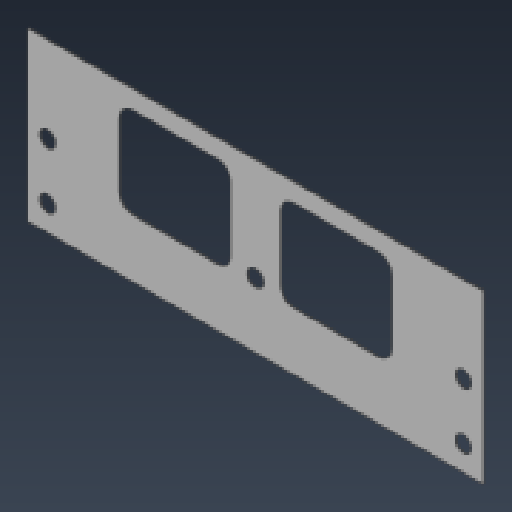
# Autodesk Inventor part: spring_steel_front
Saved by Autodesk Inventor 2023 (Build 270158000, 158)
## iProperties
Created: 2026-01-11
Part Number: spring_steel_front
Material: Steel
Document SubType Name: Modeling
Designer: szymo
Density: 7.85 g/cm^3
Appearance: Chrome - Polished
Mass: 4.02816 g
Surface Area: 52.31 cm^2
Volume: 0.513142 cm^3
Author: szymo
Autodesk Inventor part; units mm, degrees
ref_plane "YZ Plane" through (0, 0, 0) normal (1, 0, 0) x (0, 1, 0)
ref_plane "XZ Plane" through (0, 0, 0) normal (0, 1, 0) x (-1, 0, 0)
ref_plane "XY Plane" through (0, 0, 0) normal (0, 0, 1) x (1, 0, 0)
sketch "Sketch1" plane through (0, 0, 0) normal (1, 0, 0) x (0, 1, 0)
  line L0 (-35.2965, 0) -> (0, 0) projected
  line L1 (0, 0) -> (-0.5338, -2.3917) projected
  line L2 (-0.5338, -2.3917) -> (-3.9179, -1.5) projected
  line L3 (-3.9179, -1.5) -> (-35.2965, -1.5) projected
  line L4 (-35.2965, -1.5) -> (-35.2965, 0) projected
  line L5 (-35.2965, 0) -> (-35.2965, 0.2)
  line L6 (-35.2965, 0.2) -> (1.4806, 0.2)
  circle A0 centre (-31.2911, -62.214) radius 20 construction
  line L7 (-31.2911, -62.214) -> (-11.9512, -67.3099) construction
  line L8 (-11.9512, -67.3099) -> (-0.05, -2.5192) construction
  line L9 (-0.05, -2.5192) -> (1.0354, 3.3894) construction
  arc A1 (-19.5194, 0.2) -> (1.0354, 3.3894) centre (-26.178, 110.9421) ccw construction
  line L10 (-0.4577, 3.7828) -> (1.0354, 3.3894) construction
  line L11 (0, 0) -> (1.4806, 0)
  line L12 (1.4806, 0) -> (1.4806, 0.2)
  dimension "d1" = 0.2
  dimension "d2" = 21
  dimension "d3" = 15.7771
  constraints: 16 end point, 3 parallel, 2 collinear, 2 point on circle, 1 centre point, 1 coincident, 1 perpendicular, 1 point on line, 1 tangent, 5 other
  measures "d1" distance of L0.start L5.end
  measures "d2" distance of A1.start L6.end
  measures "d3" distance of L5.end A1.start
extrude "Extrusion1" add sketch "Sketch1" along normal blind 99.5 and the other way blind 0.5 contours L5 L6 L12 L11 L0
sketch "Sketch2" plane through (-0.5, -35.2965, 0.2) normal (0, 0, 1) x (1, 0, 0)
  ellipse E0 centre (37.57, 21.9101) end of major axis (37.57, 15.4967) minor radius 6.25 (37.57, 15.4967) -> (37.57, 28.3235) ccw projected
  line L0 (37.57, 15.4967) -> (27.08, 15.4967) projected
  ellipse E1 centre (27.08, 21.9101) end of major axis (27.08, 28.3235) minor radius 6.25 (27.08, 28.3235) -> (27.08, 15.4967) ccw projected
  line L1 (27.08, 28.3235) -> (37.57, 28.3235) projected
  ellipse E2 centre (72.92, 21.9101) end of major axis (72.92, 15.4967) minor radius 6.25 (72.92, 15.4967) -> (72.92, 28.3235) ccw projected
  line L2 (72.92, 15.4967) -> (62.43, 15.4967) projected
  ellipse E3 centre (62.43, 21.9101) end of major axis (62.43, 28.3235) minor radius 6.25 (62.43, 28.3235) -> (62.43, 15.4967) ccw projected
  line L3 (62.43, 28.3235) -> (72.92, 28.3235) projected
  circle A0 centre (4.25, 5.5) radius 1.8 projected
  circle A1 centre (95.75, 17.8786) radius 1.8 projected
  circle A2 centre (95.75, 5.5) radius 1.8 projected
  circle A3 centre (4.25, 17.8786) radius 1.8 projected
  circle A4 centre (50, 14.1959) radius 1.8 projected
  line L4 (99.5, 0) -> (99.5, 35.2965) projected
  line L5 (0.5, 35.2965) -> (99.5, 35.2965) projected
  line L6 (0.5, 0) -> (0.5, 35.2965) projected
  line L7 (0.5, 0) -> (99.5, 0) projected
  constraints: 4 other
extrude "Extrusion2" cut sketch "Sketch2" against normal blind 99.5 contours A0 | A1 | A2 | A3 | A4
sketch "Sketch3" plane through (-0.5, -35.2965, 0.2) normal (0, 0, 1) x (1, 0, 0)
  ellipse E0 centre (72.92, 21.9101) end of major axis (72.92, 15.4967) minor radius 6.25 (72.92, 15.4967) -> (72.92, 28.3235) ccw construction
  line L0 (62.43, 28.3235) -> (72.92, 28.3235) construction
  ellipse E1 centre (62.43, 21.9101) end of major axis (62.43, 28.3235) minor radius 6.25 (62.43, 28.3235) -> (62.43, 15.4967) ccw construction
  line L1 (72.92, 15.4967) -> (62.43, 15.4967) construction
  line L2 (37.57, 15.4967) -> (27.08, 15.4967) construction
  ellipse E2 centre (37.57, 21.9101) end of major axis (37.57, 15.4967) minor radius 6.25 (37.57, 15.4967) -> (37.57, 28.3235) ccw construction
  line L3 (27.08, 28.3235) -> (37.57, 28.3235) construction
  ellipse E3 centre (27.08, 21.9101) end of major axis (27.08, 28.3235) minor radius 6.25 (27.08, 28.3235) -> (27.08, 15.4967) ccw construction
  line L4 (74.92, 32.8235) -> (60.43, 32.8235)
  line L5 (74.92, 10.9967) -> (60.43, 10.9967)
  line L6 (39.57, 10.9967) -> (25.08, 10.9967)
  line L7 (39.57, 32.8235) -> (25.08, 32.8235)
  line L8 (79.17, 21.9101) -> (56.18, 21.9101) construction
  line L9 (74.92, 10.9967) -> (74.92, 32.8235) construction
  line L10 (60.43, 10.9967) -> (60.43, 32.8235) construction
  ellipse E4 centre (74.92, 21.9101) end of major axis (74.92, 10.9967) minor radius 6.25 (74.92, 10.9967) -> (74.92, 32.8235) ccw
  ellipse E5 centre (60.43, 21.9101) end of major axis (60.43, 10.9967) minor radius 6.25 (60.43, 32.8235) -> (60.43, 10.9967) ccw
  line L11 (43.82, 21.9101) -> (20.83, 21.9101) construction
  line L12 (39.57, 10.9967) -> (39.57, 32.8235) construction
  line L13 (25.08, 32.8235) -> (25.08, 10.9967) construction
  ellipse E6 centre (39.57, 21.9101) end of major axis (39.57, 10.9967) minor radius 6.25 (39.57, 10.9967) -> (39.57, 32.8235) ccw
  ellipse E7 centre (25.08, 21.9101) end of major axis (25.08, 10.9967) minor radius 6.25 (25.08, 32.8235) -> (25.08, 10.9967) ccw
  line L14 (79.17, 21.9101) -> (81.17, 21.9101) construction
  line L15 (56.18, 21.9101) -> (54.18, 21.9101) construction
  line L16 (43.82, 21.9101) -> (45.82, 21.9101) construction
  line L17 (20.83, 21.9101) -> (18.83, 21.9101) construction
  point P0 (0.5, 35.2965)
  dimension "d14" = 4.5
  dimension "d15" = 4.5
  dimension "d16" = 4.5
  dimension "d17" = 4.5
  dimension "d18" = 2
  dimension "d19" = 2
  dimension "d20" = 2
  dimension "d21" = 2
  dimension "d22" = 2
  dimension "d23" = 2
  dimension "d24" = 2
  dimension "d25" = 2
  dimension "d26" = 2
  dimension "d27" = 2
  dimension "d28" = 2
  dimension "d29" = 2
  constraints: 28 end point, 10 horizontal, 4 midpoint, 3 point on line, 3 vertical, 28 other
  measures "d14" distance between parallel lines of L5 L1
  measures "d15" distance between parallel lines of L0 L4
  measures "d16" distance between parallel lines of L6 L2
  measures "d17" distance between parallel lines of L7 L3
  measures "d18" horizontal distance of point (72.92, 21.91) L5.start
  measures "d19" horizontal distance of L5.end point (62.43, 21.91)
  measures "d20" horizontal distance of L4.end point (62.43, 21.91)
  measures "d21" horizontal distance of L4.start point (72.92, 21.91)
  measures "d22" horizontal distance of L6.start point (37.57, 21.91)
  measures "d23" horizontal distance of L7.start point (37.57, 21.91)
  measures "d24" horizontal distance of L7.end point (27.08, 21.91)
  measures "d25" horizontal distance of L6.end point (27.08, 21.91)
  measures "d26" distance of L8.start L14.end
  measures "d27" distance of L8.end L15.end
  measures "d28" distance of L11.start L16.end
  measures "d29" distance of L11.end L17.end
extrude "Extrusion3" [suppressed]
sketch "Sketch4" plane through (-0.5, -35.2965, 0.2) normal (0, 0, 1) x (1, 0, 0)
  ellipse E0 centre (72.92, 20.7273) end of major axis (78.17, 20.7273) minor radius 5.1162 (67.675, 20.504) -> (67.675, 20.9505) ccw construction
  ellipse E1 centre (62.43, 20.7273) end of major axis (67.68, 20.7273) minor radius 5.1162 (67.675, 20.9505) -> (67.675, 20.504) ccw construction
  ellipse E2 centre (37.57, 20.7273) end of major axis (42.82, 20.7273) minor radius 5.1162 (32.325, 20.504) -> (32.325, 20.9505) ccw construction
  ellipse E3 centre (27.08, 20.7273) end of major axis (32.33, 20.7273) minor radius 5.1162 (32.325, 20.9505) -> (32.325, 20.504) ccw construction
  line L0 (72.92, 12.7273) -> (62.43, 12.7273)
  line L1 (37.57, 12.7273) -> (27.08, 12.7273)
  line L2 (72.92, 32.7273) -> (62.43, 32.7273)
  line L3 (37.57, 32.7273) -> (27.08, 32.7273)
  line L4 (72.92, 12.7273) -> (72.92, 32.7273) construction
  line L5 (62.43, 32.7273) -> (62.43, 12.7273) construction
  line L6 (37.57, 12.7273) -> (37.57, 32.7273) construction
  line L7 (27.08, 32.7273) -> (27.08, 12.7273) construction
  circle A0 centre (76.92, 15.7273) radius 3
  circle A1 centre (58.43, 29.7273) radius 3
  circle A2 centre (41.57, 29.7273) radius 3
  circle A3 centre (41.57, 15.7273) radius 3
  circle A4 centre (23.08, 15.7273) radius 3
  circle A5 centre (23.08, 29.7273) radius 3
  circle A6 centre (76.92, 29.7273) radius 3
  circle A7 centre (58.43, 15.7273) radius 3
  line L8 (76.92, 32.7273) -> (72.92, 32.7273)
  line L9 (76.92, 12.7273) -> (72.92, 12.7273)
  line L10 (58.43, 12.7273) -> (62.43, 12.7273)
  line L11 (58.43, 32.7273) -> (62.43, 32.7273)
  line L12 (37.57, 32.7273) -> (41.57, 32.7273)
  line L13 (37.57, 12.7273) -> (41.57, 12.7273)
  line L14 (27.08, 12.7273) -> (23.08, 12.7273)
  line L15 (27.08, 32.7273) -> (23.08, 32.7273)
  line L16 (79.92, 15.7273) -> (79.92, 29.7273)
  line L17 (55.43, 15.7273) -> (55.43, 29.7273)
  line L18 (44.57, 15.7273) -> (44.57, 29.7273)
  line L19 (20.08, 15.7273) -> (20.08, 29.7273)
  line L20 (62.43, 20.7273) -> (72.92, 20.7273) construction
  line L21 (37.57, 20.7273) -> (27.08, 20.7273) construction
  line L22 (58.43, 15.7273) -> (55.43, 15.7273) construction
  line L23 (58.43, 29.7273) -> (55.43, 29.7273) construction
  line L24 (76.92, 15.7273) -> (79.92, 15.7273) construction
  line L25 (76.92, 29.7273) -> (79.92, 29.7273) construction
  line L26 (76.92, 29.7273) -> (76.92, 32.7273) construction
  line L27 (76.92, 15.7273) -> (76.92, 12.7273) construction
  line L28 (58.43, 15.7273) -> (58.43, 12.7273) construction
  line L29 (58.43, 29.7273) -> (58.43, 32.7273) construction
  line L30 (41.57, 15.7273) -> (41.57, 12.7273) construction
  line L31 (41.57, 15.7273) -> (44.57, 15.7273) construction
  line L32 (41.57, 29.7273) -> (44.57, 29.7273) construction
  line L33 (41.57, 29.7273) -> (41.57, 32.7273) construction
  line L34 (23.08, 15.7273) -> (20.08, 15.7273) construction
  line L35 (23.08, 15.7273) -> (23.08, 12.7273) construction
  line L36 (23.08, 29.7273) -> (23.08, 32.7273) construction
  line L37 (23.08, 29.7273) -> (20.08, 29.7273) construction
  point P0 (0.5, 35.2965)
  dimension "d30" = 6
  dimension "d31" = 6
  dimension "d32" = 6
  dimension "d33" = 6
  dimension "d34" = 6
  dimension "d35" = 6
  dimension "d36" = 6
  dimension "d38" = 6
  dimension "d40" = 4
  dimension "d41" = 4
  dimension "d42" = 4
  dimension "d43" = 4
  dimension "d44" = 4
  dimension "d45" = 4
  dimension "d46" = 4
  dimension "d47" = 4
  dimension "d48" = 8
  dimension "d49" = 12
  dimension "d50" = 8
  constraints: 76 end point, 16 point on circle, 16 tangent, 8 centre point, 8 horizontal, 8 point on line, 7 vertical, 6 parallel, 3 collinear, 3 perpendicular, 4 other
  measures "d30" diameter of A0
  measures "d31" diameter of A1
  measures "d32" diameter of A2
  measures "d33" diameter of A3
  measures "d34" diameter of A4
  measures "d35" diameter of A5
  measures "d36" diameter of A6
  measures "d38" diameter of A7
  measures "d40" distance of L9.start L0.start
  measures "d41" distance of L10.start L0.end
  measures "d42" distance of L8.start L2.start
  measures "d43" distance of L11.start L2.end
  measures "d44" distance of L3.start L12.end
  measures "d45" distance of L3.end L15.end
  measures "d46" distance of L1.end L14.end
  measures "d47" distance of L1.start L13.end
  measures "d48" distance between parallel lines of L0 L20
  measures "d49" distance between parallel lines of L2 L20
  measures "d50" distance between parallel lines of L1 L21
extrude "Extrusion4" cut sketch "Sketch4" against normal blind 10
equation "\"d15\" = d14"
equation "\"d16\" = d14"
equation "\"d17\" = d14"
equation "\"d19\" = d18"
equation "\"d20\" = d18"
equation "\"d21\" = d18"
equation "\"d22\" = d18"
equation "\"d23\" = d18"
equation "\"d24\" = d18"
equation "\"d25\" = d18"
equation "\"d26\" = d18"
equation "\"d27\" = d18"
equation "\"d28\" = d18"
equation "\"d29\" = d18"
equation "\"d31\" = d37"
equation "\"d32\" = d30"
equation "\"d33\" = d30"
equation "\"d34\" = d30"
equation "\"d35\" = d30"
equation "\"d36\" = d37"
equation "\"d38\" = d37"
equation "\"d41\" = d40"
equation "\"d42\" = d40"
equation "\"d43\" = d40"
equation "\"d44\" = d40"
equation "\"d45\" = d40"
equation "\"d46\" = d40"
equation "\"d47\" = d40"
equation "\"d50\" = d48"
equation "\"d37\" = 6"
body "Solid1"
